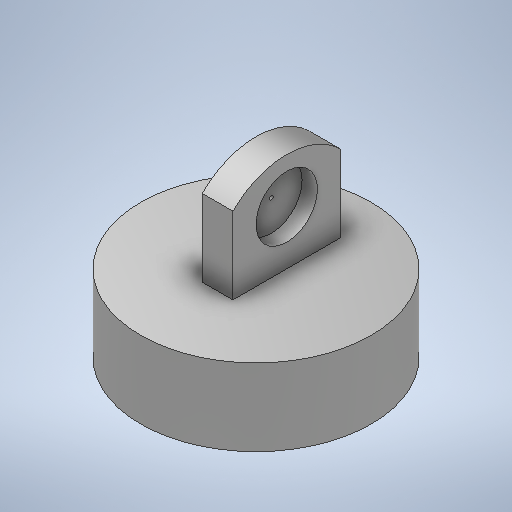
# Autodesk Inventor part: Robot_arm_base
Saved by Autodesk Inventor 2025 (Build 290162010, 162A)
## iProperties
Created: 2024-07-13
Part Number: Robot_arm_base
Material: Generic
Document SubType Name: Modeling
Designer: saees
Density: 1 g/cm^3
Appearance: Anodized - Light Gray
Author: saees
Autodesk Inventor part; units mm, degrees
ref_plane "YZ Plane" through (0, 0, 0) normal (1, 0, 0) x (0, 1, 0)
ref_plane "XZ Plane" through (0, 0, 0) normal (0, 1, 0) x (-1, 0, 0)
ref_plane "XY Plane" through (0, 0, 0) normal (0, 0, 1) x (1, 0, 0)
sketch "Sketch1" plane through (0, 0, 0) normal (0, 1, 0) x (-1, 0, 0)
  circle A0 centre (0, 0) radius 150
  dimension "d0" = 300
  constraints: 1 centre point, 1 coincident
  measures "d0" diameter of A0
extrude "Extrusion1" add sketch "Sketch1" along normal blind 100
sketch "Sketch2" plane through (0, 100, 0) normal (0, 1, 0) x (1, 0, 0)
  line L0 (-20, -50) -> (20, -50)
  line L1 (20, -50) -> (20, 90)
  line L2 (20, 90) -> (-20, 90)
  line L3 (-20, 90) -> (-20, -50)
  point P0 (0, 0)
  dimension "d3" = 140
  dimension "d4" = 40
  dimension "d5" = 50
  dimension "d6" = 20
  constraints: 8 end point, 2 parallel, 1 horizontal, 1 perpendicular
  measures "d3" distance of L2.end L0.start
  measures "d4" distance of L0.start L0.end
  measures "d5" distance from line of L0 point (0, 0)
  measures "d6" horizontal distance of point (0, 0) L0.start
extrude "Extrusion2" add sketch "Sketch2" along normal blind 100
sketch "Sketch3" plane through (20, 100, 50) normal (1, 0, 0) x (0, 0, -1)
  line L0 (0, 100) -> (140, 100) projected
  arc A0 (140, 100) -> (0, 100) centre (70, 29.7912) ccw
  line L1 (0, 0) -> (0, 100) projected
  line L2 (0, 100) -> (140, 100)
  point P0 (50, -100)
  dimension "d9" = 99.1427
  constraints: 2 end point, 2 point on circle, 1 centre point, 1 point on line
  measures "d9" radius of A0
extrude "Extrusion3" add sketch "Sketch3" against normal blind 40
sketch "Sketch4" plane through (20, 100, 50) normal (1, 0, 0) x (0, 0, -1)
  circle A0 centre (70, 70) radius 40
  line L0 (200, 0) -> (-100, 0) projected
  line L1 (0, 0) -> (0, 100) projected
  point P0 (50, -100)
  dimension "d12" = 80
  dimension "d13" = 70
  dimension "d14" = 70
  constraints: 1 centre point
  measures "d12" diameter of A0
  measures "d13" distance from line of L0 A0.centre
  measures "d14" distance from line of L1 A0.centre
extrude "Extrusion4" cut sketch "Sketch4" against normal blind 20
sketch "Sketch5" plane through (0, 170, -20) normal (1, 0, 0) x (0, 0, -1)
  circle A0 centre (0, 0) radius 2.5
  circle A1 centre (0, 0) radius 40 projected
  point P0 (-20, -170)
  dimension "d20" = 5
  constraints: 2 coincident, 1 centre point
  measures "d20" diameter of A0
extrude "Extrusion5" cut sketch "Sketch5" against normal blind 20 contours A0
sketch "Sketch6" plane through (0, 0, 0) normal (0, -1, 0) x (1, 0, 0)
  line L0 (-20, 50) -> (-20, -90) projected
  line L1 (20, -90) -> (20, 50) projected
  line L2 (20, 50) -> (-20, 50) projected
  line L3 (-20, -90) -> (20, -90) projected
  line L4 (-15, 15) -> (15, 15)
  line L5 (15, 15) -> (15, -55)
  line L6 (15, -55) -> (-15, -55)
  line L7 (-15, -55) -> (-15, 15)
  point P0 (0, 0)
  point P1 (0, 15)
  point P2 (0, 50)
  point P3 (15, -20)
  point P4 (20, -20)
  dimension "d23" = 30
  dimension "d24" = 70
  constraints: 8 end point, 4 midpoint, 2 parallel, 1 horizontal, 1 horizontal alignment, 1 perpendicular, 1 vertical alignment
  measures "d23" distance of L4.start L4.end
  measures "d24" distance of L6.end L4.start
extrude "Extrusion6" cut sketch "Sketch6" against normal blind 90 contours L4 L5 L6 L7
sketch "Sketch7" plane through (0, 90, 0) normal (0, -1, 0) x (1, 0, 0)
  line L0 (15, -55) -> (-15, -55) projected
  line L1 (15, 15) -> (15, -55) projected
  line L2 (-15, 15) -> (15, 15) projected
  line L3 (-15, -55) -> (-15, 15) projected
  line L4 (0, 20) -> (0, -60) projected
  circle A0 centre (0, -20) radius 2.5
  point P0 (0, 0)
  dimension "d28" = 5
  constraints: 1 centre point, 1 midpoint
  measures "d28" diameter of A0
extrude "Extrusion7" cut sketch "Sketch7" against normal blind 30 contours A0 L4 | L4 A0
body "Solid1"
